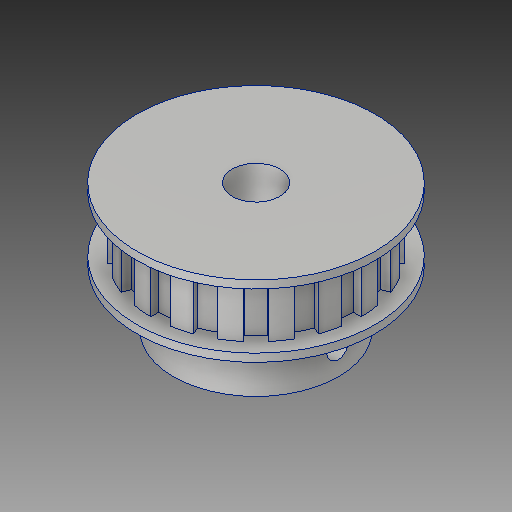
# Autodesk Inventor part: LargeBelt_Pulley
Saved by Autodesk Inventor 2019.4 (Build 234330000, 330)
## iProperties
Created: 2021-02-01
Part Number: LargeBelt_Pulley
Material: Generic
Document SubType Name: Modeling
Designer: Jorian Brusind
Density: 1 g/cm^3
Appearance: Aluminum - Flat
Mass: 54.5642 g
Surface Area: 144.49 cm^2
Volume: 54.5642 cm^3
Author: Jorian Brusind
Autodesk Inventor part; units mm, degrees
ref_plane "YZ Plane" through (0, 0, 0) normal (1, 0, 0) x (0, 1, 0)
ref_plane "XZ Plane" through (0, 0, 0) normal (0, 1, 0) x (-1, 0, 0)
ref_plane "XY Plane" through (0, 0, 0) normal (0, 0, 1) x (1, 0, 0)
sketch "Sketch1" plane through (0, 0, 0) normal (0, 1, 0) x (-1, 0, 0)
  circle A0 centre (0, 0) radius 20.75
  dimension "d0" = 41.5
  constraints: 1 centre point, 1 coincident
  measures "d0" diameter of A0
extrude "Extrusion1" add sketch "Sketch1" along normal blind 32
sketch "Sketch2" plane through (0, 32, 0) normal (0, 1, 0) x (1, 0, 0)
  circle A0 centre (0, 0) radius 30
  dimension "d3" = 60
  constraints: 1 centre point, 1 coincident
  measures "d3" diameter of A0
extrude "Extrusion2" add sketch "Sketch2" against normal blind 18
sketch "Sketch3" plane through (0, 0, 0) normal (1, 0, 0) x (0, 1, 0)
  line L0 (32, 30) -> (32, -30) projected
  line L1 (32, -30) -> (30, -30)
  line L2 (32, -30) -> (14, -30) projected
  line L3 (30, -30) -> (30, -24.5)
  line L4 (14, 30) -> (14, -30) projected
  line L5 (14, -30) -> (16, -30)
  line L6 (16, -30) -> (16, -24.5)
  line L7 (16, -24.5) -> (30, -24.5)
  line L8 (16, -30) -> (30, -30)
  line L9 (0, 0) -> (32, 0)
  dimension "d6" = 2
  dimension "d7" = 5.5
  dimension "d8" = 2
  constraints: 14 end point, 2 perpendicular, 2 point on line, 1 midpoint, 1 parallel, 1 vertical
  measures "d6" distance of L0.end L1.end
  measures "d7" distance of L1.end L3.end
  measures "d8" distance of L2.end L5.end
revolve "Revolution1" cut sketch "Sketch3" angle 360 about axis through (0, 0, 0) along (0, 1, 0) contours L2 L6 L7 L3
sketch "Sketch4" plane through (0, 0, 0) normal (1, 0, 0) x (0, 1, 0)
  line L0 (16, -24.5) -> (30, -24.5) projected
  line L1 (16, -24.5) -> (30, -24.5)
  line L2 (16, -24.5) -> (16, -26.5)
  line L3 (16, 30) -> (16, -30) projected
  line L4 (16, -26.5) -> (30, -26.5)
  line L5 (30, -24.5) -> (30, -26.5)
  line L6 (30, -30) -> (30, 30) projected
  line L7 (32, 30) -> (32, -30) projected
  line L8 (0, 0) -> (32, 0)
  dimension "d10" = 2
  dimension "d11" = 2
  constraints: 10 end point, 3 point on line, 1 collinear, 1 midpoint, 1 perpendicular
  measures "d10" distance of L0.start L2.end
  measures "d11" distance between parallel lines of L7 L5
revolve "Revolution2" add sketch "Sketch4" angle 10 about axis through (0, 0, 0) along (0, -1, 0) contours L0 L5 L4 L2
pattern_circular "Circular Pattern1" count 18 over 360 about axis through (0, 23, 0) along (0, -1, 0) of "Revolution2"
sketch "Sketch5" plane through (0, 0, 0) normal (0, -1, 0) x (1, 0, 0)
  circle A0 centre (0, 0) radius 6
  dimension "d16" = 12
  constraints: 1 centre point, 1 coincident
  measures "d16" diameter of A0
extrude "Extrusion3" cut sketch "Sketch5" against normal up to next
sketch "Sketch6" plane through (0, 0, 0) normal (1, 0, 0) x (0, 1, 0)
  line L0 (0, 0) -> (6.5, 0)
  circle A0 centre (6.5, 0) radius 2.75
  dimension "d19" = 6.5
  dimension "d20" = 5.5
  constraints: 2 end point, 1 centre point, 1 coincident, 1 horizontal
  measures "d19" distance of L0.start L0.end
  measures "d20" diameter of A0
extrude "Extrusion4" cut sketch "Sketch6" along normal up to surface
pattern_circular "Circular Pattern2" count 2 over 90 about axis through (0, 0, 0) along (0, 1, 0) of "Extrusion4"
body "Solid1"
